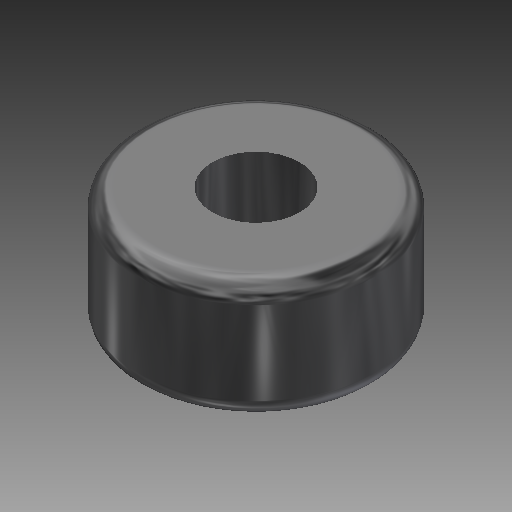
# Autodesk Inventor part: Gommino inferiore
Saved by Autodesk Inventor 2019 (Build 230136000, 136)
## iProperties
Created: 2011-09-21
Part Number: Gommino inferiore
Document SubType Name: Modeling
Designer: Stefano
Density: 1 g/cm^3
Material: 一般
Appearance: ゴム - 黒 - バージョン 1.1
Author: Stefano
Autodesk Inventor part; units mm, degrees
ref_plane "YZ Plane" through (0, 0, 0) normal (1, 0, 0) x (0, 1, 0)
ref_plane "XZ Plane" through (0, 0, 0) normal (0, 1, 0) x (-1, 0, 0)
ref_plane "XY Plane" through (0, 0, 0) normal (0, 0, 1) x (1, 0, 0)
sketch "Schizzo1" plane through (0, 0, 0) normal (0, 0, 1) x (1, 0, 0)
  line L0 (4.75, 6.5) -> (4.75, -6.5)
  line L1 (13, -4.5) -> (13, 4.5)
  line L2 (11, 6.5) -> (4.75, 6.5)
  line L3 (4.75, -6.5) -> (11, -6.5)
  arc A0 (11, -6.5) -> (13, -4.5) centre (11, -4.5) ccw
  arc A1 (13, 4.5) -> (11, 6.5) centre (11, 4.5) ccw
  line L4 (0, -9.6799) -> (0, 9.6799) projected
  point P0 (0, 0)
  point P1 (13, -6.5)
  point P2 (13, 6.5)
  dimension "d2" = 13
  dimension "d3" = 2
  constraints: 8 end point, 4 point on circle, 4 point on line, 4 tangent, 2 centre point, 2 parallel, 1 equal radius, 1 perpendicular
  measures "d2" distance of point (13, -6.5) point (13, 6.5)
  measures "d3" radius of A0
revolve "Rivoluzione1" add sketch "Schizzo1" angle 360 about axis through (0, -10, 0) along (0, 1, 0)
